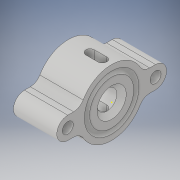
# Autodesk Inventor part: output
Saved by Autodesk Inventor 2018 (Build 220112000, 112)
## iProperties
Created: 2020-03-28
Part Number: output
Material: Generic
Document SubType Name: Modeling
Designer: emile
Density: 1 g/cm^3
Appearance: Default
Author: emile
Title: OUTPUT
Autodesk Inventor part; units mm, degrees
ref_plane "YZ Plane" through (0, 0, 0) normal (1, 0, 0) x (0, 1, 0)
ref_plane "XZ Plane" through (0, 0, 0) normal (0, 1, 0) x (-1, 0, 0)
ref_plane "XY Plane" through (0, 0, 0) normal (0, 0, 1) x (1, 0, 0)
sketch "Sketch2" plane through (0, 0, 0) normal (0, 0, 1) x (1, 0, 0)
  line L0 (-28.55236, 19.05) -> (28.55236, 19.05)
  line L1 (28.55236, 19.05) -> (28.55236, 0)
  line L2 (28.55236, 0) -> (-28.55236, 0)
  line L3 (-28.55236, 0) -> (-28.55236, 19.05)
  line L4 (-6.228741, 5.715) -> (-3.498241, 8.4455)
  line L5 (-6.228741, 5.715) -> (-28.55236, 5.715)
  line L6 (-3.498241, 8.4455) -> (0, 8.4455)
  line L7 (0, 8.4455) -> (0, 0)
  line L8 (0, 8.4455) -> (0, 19.05)
  circle A0 centre (0, 0) radius 7.9375 construction
  line L9 (-2.208873, 9.016447) -> (-4.364135, 6.861186) construction
  circle A1 centre (-3.498241, 14.2875) radius 1.524
  line L10 (-7.59736, 2.2987) -> (-28.55236, 2.2987) construction
  line L11 (-25.37736, 5.715) -> (-25.37736, 2.2987)
  line L12 (-25.37736, 0) -> (-25.37736, 2.2987)
  line L13 (-15.85236, 5.715) -> (-15.85236, 2.2987)
  line L14 (-15.85236, 2.54) -> (-25.37736, 2.54)
  line L15 (-3.498241, 8.4455) -> (-3.498241, 19.05)
  dimension "d37" = 15.875
  dimension "d10" = 19.05
  dimension "d35" = 45
  dimension "d36" = 0.508
  dimension "d38" = 5.715
  dimension "d39" = 8.4455
  dimension "d40" = 3.048
  dimension "d41" = 14.2875
  dimension "d43" = 2.2987
  dimension "d44" = 20.955
  dimension "d45" = 3.175
  dimension "d46" = 9.525
  dimension "d47" = 2.54
  constraints: 32 end point, 11 point on line, 7 perpendicular, 3 parallel, 2 coincident, 2 horizontal, 2 midpoint, 1 centre point, 1 collinear, 1 vertical, 1 vertical alignment, 4 other
  measures "d10" distance between parallel lines of L2 L0
  measures "d35" angle of L6 L4
  measures "d36" distance between parallel lines of L4 L9
  measures "d38" distance between parallel lines of L2 L5
  measures "d39" distance between parallel lines of L2 L6
  measures "d40" diameter of A1
  measures "d41" distance from line of L2 A1.centre
  measures "d43" distance between parallel lines of L2 L10
  measures "d44" distance of L10.start L10.end
  measures "d45" distance between parallel lines of L3 L11
  measures "d46" distance between parallel lines of L11 L13
  measures "d47" distance between parallel lines of L2 L14
sketch "Sketch2 outline for Revolution1" plane through (0, 0, 0) normal (0, 0, 1) x (1, 0, 0)
  line L0 (-28.55236, 0) -> (-25.37736, 0)
  line L1 (-25.37736, 0) -> (-25.37736, 2.54)
  line L2 (-25.37736, 2.54) -> (-15.85236, 2.54)
  line L3 (-15.85236, 2.54) -> (-15.85236, 5.715)
  line L4 (-15.85236, 5.715) -> (-6.228741, 5.715)
  line L5 (-6.228741, 5.715) -> (-3.498241, 8.4455)
  line L6 (-3.498241, 8.4455) -> (-3.498241, 19.05)
  line L7 (-3.498241, 19.05) -> (-28.55236, 19.05)
  line L8 (-28.55236, 19.05) -> (-28.55236, 0)
revolve "Revolution1" add sketch "Sketch2 outline for Revolution1" angle 360 about axis through (28.55236, 0, 0) along (-1, 0, 0)
sketch "Sketch2 outline for Revolution2" plane through (0, 0, 0) normal (0, 0, 1) x (1, 0, 0)
  circle A0 centre (-3.498241, 14.2875) radius 1.524
revolve "Revolution2" cut sketch "Sketch2 outline for Revolution2" angle 360 about axis through (28.55236, 0, 0) along (-1, 0, 0)
sketch "Sketch5" plane through (-15.85236, 0, 0) normal (1, 0, 0) x (0, 0, -1)
  circle A0 centre (0, 0) radius 5.715
  circle A1 centre (0, 0) radius 2.54
  circle A2 centre (0, 4.064) radius 0.79375
  point P0 (0, 0)
  dimension "d48" = 1.5875
  dimension "d49" = 4.064
  constraints: 1 centre point, 1 vertical alignment
  measures "d48" diameter of A2
  measures "d49" distance of A2.centre point (0, 0)
sketch "Sketch5 outline for Extrusion4" plane through (-15.85236, 0, 0) normal (1, 0, 0) x (0, 0, -1)
  circle A0 centre (0, 4.064) radius 0.79375
extrude "Extrusion4" cut sketch "Sketch5 outline for Extrusion4" against normal through all
pattern_circular "Circular Pattern2" count 10 over 360 about axis through (-20.61486, 0, 0) along (1, 0, 0) of "Extrusion4"
sketch "Sketch6" plane through (0, 0, 0) normal (0, 1, 0) x (-1, 0, 0)
  line L0 (6.228741, 5.715) -> (6.228741, -5.715)
  line L1 (15.85236, 5.715) -> (15.85236, -5.715)
  line L2 (15.85236, 2.54) -> (15.85236, -2.54)
  line L3 (25.37736, 2.54) -> (25.37736, -2.54)
  line L4 (22.83736, 0) -> (8.768741, 0) construction
  line L5 (22.83736, -2.54) -> (8.768741, -2.54)
  line L6 (8.768741, 2.54) -> (22.83736, 2.54)
  arc A0 (22.83736, -2.54) -> (22.83736, 2.54) centre (22.83736, 0) ccw
  arc A1 (8.768741, 2.54) -> (8.768741, -2.54) centre (8.768741, 0) ccw
  circle A2 centre (15.803051, 0) radius 2.54
  line L7 (15.803051, 0) -> (8.768741, 0) construction
  line L8 (15.803051, 2.54) -> (8.768741, 2.54)
  line L9 (8.768741, -2.54) -> (15.803051, -2.54)
  arc A3 (15.803051, -2.54) -> (15.803051, 2.54) centre (15.803051, 0) ccw
  arc A4 (8.768741, 2.54) -> (8.768741, -2.54) centre (8.768741, 0) ccw
  point P0 (0, 0)
  point P1 (12.285896, 0)
  point P2 (6.228741, 0)
  constraints: 16 end point, 12 tangent, 10 point on circle, 5 centre point, 2 horizontal, 2 horizontal alignment, 2 midpoint, 2 parallel, 1 coincident
sketch "Sketch6 outline for Extrusion5" plane through (0, 0, 0) normal (0, 1, 0) x (-1, 0, 0)
  arc A0 (15.803051, -2.54) -> (15.803051, 2.54) centre (15.803051, 0) ccw
  line L0 (8.768741, -2.54) -> (15.803051, -2.54)
  arc A1 (6.228741, 0) -> (8.768741, -2.54) centre (8.768741, 0) ccw
  arc A2 (8.768741, 2.54) -> (6.228741, 0) centre (8.768741, 0) ccw
  line L1 (15.803051, 2.54) -> (8.768741, 2.54)
extrude "Extrusion5" cut sketch "Sketch6 outline for Extrusion5" along normal through all both and the other way through all
sketch "Sketch7" plane through (-15.85236, 0, 0) normal (1, 0, 0) x (0, 0, -1)
  arc A0 (2.539521, 2.508544) -> (2.539521, 4.067146) centre (2.388759, 3.287845) ccw
  circle A1 centre (3.865094, 1.255845) radius 0.79375
  circle A2 centre (3.865094, -1.255845) radius 0.79375
  arc A3 (2.539521, -4.067146) -> (2.539521, -2.508544) centre (2.388759, -3.287845) ccw
  arc A4 (-2.539521, -2.508544) -> (-2.539521, -4.067146) centre (-2.388759, -3.287845) ccw
  circle A5 centre (-3.865094, -1.255845) radius 0.79375
  circle A6 centre (-3.865094, 1.255845) radius 0.79375
  arc A7 (-2.539521, 4.067146) -> (-2.539521, 2.508544) centre (-2.388759, 3.287845) ccw
  arc A8 (-2.539521, 5.119771) -> (-2.539521, -5.119771) centre (0, 0) ccw
  arc A9 (2.539521, -5.119771) -> (2.539521, 5.119771) centre (0, 0) ccw
  spline S0 degree 2 poles (0.79375, 4.064) (0.79375, 5.438815) (-0.396875, 4.751408) (-1.5875, 4.064) (-0.396875, 3.376592) (0.79375, 2.689185) (0.79375, 4.064) knots 0 0 0 0.33333333 0.33333333 0.66666667 0.66666667 1 1 1 weights 1 0.5 1 0.5 1 0.5 1
  line L0 (-2.54, -5.119534) -> (-2.54, -18.879907)
  line L1 (-2.54, 18.879907) -> (-2.54, 5.119534)
  arc A10 (2.539521, 0.04931) -> (-2.539521, 0.04931) centre (0, 0) ccw
  line L2 (2.54, -18.879907) -> (2.54, -5.119534)
  line L3 (2.54, 5.119534) -> (2.54, 18.879907)
  line L4 (2.54, -18.879907) -> (2.54, -5.119534)
  line L5 (2.54, 5.119534) -> (2.54, 18.879907)
  arc A11 (-2.539521, -0.04931) -> (2.539521, -0.04931) centre (0, 0) ccw
  line L6 (-2.54, -5.119534) -> (-2.54, -18.879907)
  line L7 (-2.54, 18.879907) -> (-2.54, 5.119534)
  spline S1 degree 2 poles (-0.79375, -4.064) (-0.79375, -5.438815) (0.396875, -4.751408) (1.5875, -4.064) (0.396875, -3.376592) (-0.79375, -2.689185) (-0.79375, -4.064) knots 0 0 0 0.33333333 0.33333333 0.66666667 0.66666667 1 1 1 weights 1 0.5 1 0.5 1 0.5 1
  arc A12 (0, -5.715) -> (0, 5.715) centre (0, 0) ccw
  arc A13 (0, 5.715) -> (0, -5.715) centre (0, 0) ccw
  line L8 (-2.539521, 5.119771) -> (-2.54, 5.119534)
  line L9 (-2.539521, 4.067146) -> (-2.539521, 5.119771)
  line L10 (-2.539521, 0.04931) -> (-2.539521, 2.508544)
  arc A14 (2.539521, 0.04931) -> (-2.539521, 0.04931) centre (0, 0) ccw
  line L11 (2.539521, 2.508544) -> (2.539521, 0.04931)
  line L12 (2.539521, 5.119771) -> (2.539521, 4.067146)
  line L13 (2.54, 5.119534) -> (2.539521, 5.119771)
  line L14 (2.539521, -5.119771) -> (2.54, -5.119534)
  line L15 (2.539521, -4.067146) -> (2.539521, -5.119771)
  line L16 (2.539521, -0.04931) -> (2.539521, -2.508544)
  line L17 (-2.539521, -2.508544) -> (-2.539521, -0.04931)
  line L18 (-2.539521, -5.119771) -> (-2.539521, -4.067146)
  line L19 (-2.54, -5.119534) -> (-2.539521, -5.119771)
  line L20 (-2.539521, 5.119771) -> (-2.54, 5.119534)
  line L21 (-2.539521, 4.067146) -> (-2.539521, 5.119771)
  line L22 (-2.539521, 0.04931) -> (-2.539521, 2.508544)
  line L23 (2.539521, 2.508544) -> (2.539521, 0.04931)
  line L24 (2.539521, 5.119771) -> (2.539521, 4.067146)
  line L25 (2.54, 5.119534) -> (2.539521, 5.119771)
  line L26 (2.539521, -5.119771) -> (2.54, -5.119534)
  line L27 (2.539521, -4.067146) -> (2.539521, -5.119771)
  line L28 (2.539521, -0.04931) -> (2.539521, -2.508544)
  arc A15 (-2.539521, -0.04931) -> (2.539521, -0.04931) centre (0, 0) ccw
  line L29 (-2.539521, -2.508544) -> (-2.539521, -0.04931)
  line L30 (-2.539521, -5.119771) -> (-2.539521, -4.067146)
  line L31 (-2.54, -5.119534) -> (-2.539521, -5.119771)
  line L32 (2.539521, -4.067146) -> (2.539521, -5.119771)
  line L33 (2.539521, 5.119771) -> (2.539521, 4.067146)
  line L34 (2.539521, 2.508544) -> (2.539521, 0.04931)
  arc A16 (2.539521, -0.04931) -> (2.539521, 0.04931) centre (0, 0) ccw
  line L35 (2.539521, -0.04931) -> (2.539521, -2.508544)
  line L36 (-2.539521, -2.508544) -> (-2.539521, -0.04931)
  arc A17 (-2.539521, 0.04931) -> (-2.539521, -0.04931) centre (0, 0) ccw
  line L37 (-2.539521, 0.04931) -> (-2.539521, 2.508544)
  line L38 (-2.539521, 4.067146) -> (-2.539521, 5.119771)
  line L39 (-2.539521, -5.119771) -> (-2.539521, -4.067146)
  point P0 (0, 0)
  point P1 (2.54, -5.119534)
  point P2 (2.54, 5.119534)
  point P3 (-2.54, -5.119534)
  point P4 (-2.54, 5.119534)
  constraints: 8 vertical alignment, 4 horizontal alignment, 2 other
sketch "Sketch7 outline for Extrusion6" plane through (-15.85236, 0, 0) normal (1, 0, 0) x (0, 0, -1)
  circle A0 centre (0, 0) radius 5.715
extrude "Extrusion6" cut sketch "Sketch7 outline for Extrusion6" against normal blind 6.35
sketch "Sketch8" plane through (-25.37736, 0, 0) normal (1, 0, 0) x (0, 0, -1)
  circle A0 centre (0, 0) radius 1.905
  point P0 (0, 0)
  dimension "d59" = 3.81
  constraints: 1 centre point, 1 coincident
  measures "d59" diameter of A0
sketch "Sketch8 outline for Extrusion7" plane through (-25.37736, 0, 0) normal (1, 0, 0) x (0, 0, -1)
  circle A0 centre (0, 0) radius 1.905
extrude "Extrusion7" cut sketch "Sketch8 outline for Extrusion7" against normal through all
sketch "Sketch9" plane through (-3.498241, 0, 0) normal (1, 0, 0) x (0, 0, -1)
  point P0 (0, 0)
sketch "Sketch10" plane through (-3.498241, 0, 0) normal (1, 0, 0) x (0, 0, -1)
  line L0 (-25.4, 6.35) -> (-17.960512, 6.35)
  arc A0 (-25.4, 6.35) -> (-25.4, -6.35) centre (-25.4, 0) ccw
  line L1 (-25.4, -6.35) -> (-17.960512, -6.35)
  circle A1 centre (-25.4, 0) radius 1.5875
  circle A2 centre (0, 0) radius 19.05
  point P0 (0, 0)
sketch "Sketch10 outline for Extrusion8" plane through (-3.498241, 0, 0) normal (1, 0, 0) x (0, 0, -1)
  line L0 (-17.960512, 6.35) -> (-25.4, 6.35)
  arc A0 (-17.960512, -6.35) -> (-17.960512, 6.35) centre (0, 0) cw
  arc A1 (-25.4, 6.35) -> (-25.4, -6.35) centre (-25.4, 0) ccw
  line L1 (-25.4, -6.35) -> (-17.960512, -6.35)
  circle A2 centre (-25.4, 0) radius 1.5875
extrude "Extrusion8" add sketch "Sketch10 outline for Extrusion8" against normal up to surface (25.05412 mm away)
fillet "Fillet3" radius 6.35 2 edges at (-16.0253, -6.35, 17.9605) (-16.0253, 6.35, 17.9605)
pattern_circular "Circular Pattern3" count 2 over 360 about axis through (-16.025301, 0, 0) along (1, 0, 0) of "Extrusion8", "Fillet3"
sketch "Sketch11" plane through (-3.498241, 0, 25.4) normal (1, 0, 0) x (0, 0, -1)
  circle A0 centre (50.8, 0) radius 1.5875
  circle A1 centre (0, 0) radius 1.5875
  circle A2 centre (25.4, 0) radius 15.8115
  arc A3 (8.902216, -9.525) -> (41.897784, -9.525) centre (25.4, 0) ccw
  arc A4 (47.397045, -6.35) -> (41.897784, -9.525) centre (47.397045, -12.7) ccw
  line L0 (47.397045, -6.35) -> (50.8, -6.35)
  arc A5 (50.8, -6.35) -> (50.8, 6.35) centre (50.8, 0) ccw
  line L1 (50.8, 6.35) -> (47.397045, 6.35)
  arc A6 (41.897784, 9.525) -> (47.397045, 6.35) centre (47.397045, 12.7) ccw
  arc A7 (41.897784, 9.525) -> (8.902216, 9.525) centre (25.4, 0) ccw
  arc A8 (3.402955, 6.35) -> (8.902216, 9.525) centre (3.402955, 12.7) ccw
  line L2 (3.402955, 6.35) -> (0, 6.35)
  arc A9 (0, 6.35) -> (0, -6.35) centre (0, 0) ccw
  line L3 (0, -6.35) -> (3.402955, -6.35)
  arc A10 (8.902216, -9.525) -> (3.402955, -6.35) centre (3.402955, -12.7) ccw
  circle A11 centre (0, 0) radius 3.175
  circle A12 centre (50.8, 0) radius 3.175
  point P0 (25.4, 0)
  dimension "d69" = 6.35
  constraints: 2 centre point, 2 coincident, 1 equal radius
  measures "d69" diameter of A11
sketch "Sketch11 outline for Extrusion9" plane through (-3.498241, 0, 25.4) normal (1, 0, 0) x (0, 0, -1)
  circle A0 centre (0, 0) radius 3.175
  circle A1 centre (0, 0) radius 1.5875
  circle A2 centre (50.8, 0) radius 3.175
  circle A3 centre (50.8, 0) radius 1.5875
extrude "Extrusion9" cut sketch "Sketch11 outline for Extrusion9" against normal through all
body "Solid2"
